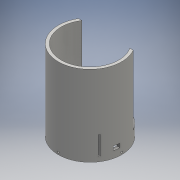
# Autodesk Inventor part: outsideCover
Saved by Autodesk Inventor 2016 (Build 200138000, 138)
## iProperties
Created: 2016-10-27
Part Number: outsideCover
Material: 一般
Document SubType Name: Modeling
Designer: Daisuke
Density: 1 g/cm^3
Appearance: 既定
Author: Daisuke
Autodesk Inventor part; units mm, degrees
ref_plane "XY Plane" through (0, 0, 0) normal (0, 0, 1) x (1, 0, 0)
sketch "スケッチ1" plane through (0, 0, 0) normal (0, 0, 1) x (1, 0, 0)
  circle A0 centre (0, 0) radius 50
  circle A1 centre (0, 0) radius 55
  line L0 (0, 0) -> (47.6314, 27.5) construction
  line L1 (0, 0) -> (55, 0) construction
  line L2 (0, 0) -> (-47.6314, 27.5) construction
  line L3 (0, 0) -> (55, 0) construction
  dimension "d0" = 100
  dimension "d1" = 110
  dimension "d2" = 30
  dimension "d3" = 150
  constraints: 8 end point, 2 centre point, 2 coincident, 2 equal length, 2 horizontal, 2 point on circle
  measures "d0" diameter of A0
  measures "d1" diameter of A1
  measures "d2" angle of L1 L0
  measures "d3" angle of L3 L2
extrude "押し出し1" add sketch "スケッチ1" along normal blind 20
sketch "スケッチ2" plane through (0, 0, 20) normal (0, 0, 1) x (1, 0, 0)
  arc A0 (-41.7582, 27.5) -> (41.7582, 27.5) centre (0, 0) ccw
  arc A1 (-47.6314, 27.5) -> (47.6314, 27.5) centre (0, 0) ccw
  line L0 (0, 0) -> (47.6314, 27.5) construction
  circle A2 centre (0, 0) radius 55 construction
  line L1 (0, 0) -> (55, 0) construction
  line L2 (0, 0) -> (-47.6314, 27.5) construction
  line L3 (0, 0) -> (55, 0) construction
  line L4 (-47.6314, 27.5) -> (-41.7582, 27.5)
  line L5 (41.7582, 27.5) -> (47.6314, 27.5)
  dimension "d6" = 30
  dimension "d7" = 150
  constraints: 12 end point, 6 point on circle, 2 centre point, 2 coincident, 2 equal length, 2 horizontal
  measures "d6" angle of L1 L0
  measures "d7" angle of L3 L2
extrude "押し出し2" add sketch "スケッチ2" along normal blind 120
ref_plane "作業平面1" through (55, 0, 0) normal (1, 0, 0) x (0, 1, 0)
ref_plane "作業平面2" through (-55, 0, 0) normal (1, 0, 0) x (0, 1, 0)
ref_plane "作業平面3" through (0, 55, 0) normal (0, 1, 0) x (-1, 0, 0)
ref_plane "作業平面4" through (0, -55, 0) normal (0, 1, 0) x (-1, 0, 0)
sketch "スケッチ3" plane through (55, 0, 0) normal (1, 0, 0) x (0, 1, 0)
  line L0 (0, 0) -> (0, 4) construction
  circle A0 centre (0, 4) radius 1.5
  dimension "d14" = 4
  dimension "d15" = 3
  constraints: 2 end point, 1 centre point, 1 coincident, 1 vertical
  measures "d14" distance of L0.start L0.end
  measures "d15" diameter of A0
extrude "押し出し3" cut sketch "スケッチ3" against normal blind 6
sketch "スケッチ4" plane through (0, 55, 0) normal (0, 1, 0) x (-1, 0, 0)
  line L0 (0, 0) -> (0, 4) construction
  circle A0 centre (0, 4) radius 1.5
  dimension "d18" = 4
  dimension "d19" = 3
  constraints: 2 end point, 1 centre point, 1 coincident, 1 vertical
  measures "d18" distance of L0.start L0.end
  measures "d19" diameter of A0
extrude "押し出し4" cut sketch "スケッチ4" against normal blind 6
sketch "スケッチ5" plane through (-55, 0, 0) normal (1, 0, 0) x (0, 1, 0)
  line L0 (0, 0) -> (0, 4) construction
  circle A0 centre (0, 4) radius 1.5
  dimension "d22" = 4
  dimension "d23" = 3
  constraints: 2 end point, 1 centre point, 1 coincident, 1 vertical
  measures "d22" distance of L0.start L0.end
  measures "d23" diameter of A0
extrude "押し出し5" cut sketch "スケッチ5" along normal blind 6
sketch "スケッチ6" plane through (0, -55, 0) normal (0, 1, 0) x (-1, 0, 0)
  line L0 (0, 0) -> (0, 4) construction
  circle A0 centre (0, 4) radius 1.5
  dimension "d26" = 4
  dimension "d27" = 3
  constraints: 2 end point, 1 centre point, 1 coincident, 1 vertical
  measures "d26" distance of L0.start L0.end
  measures "d27" diameter of A0
extrude "押し出し6" cut sketch "スケッチ6" along normal blind 6
ref_plane "作業平面5" through (55, 0, 0) normal (1, 0, 0) x (0, 1, 0)
sketch "スケッチ7" plane through (55, 0, 0) normal (1, 0, 0) x (0, 1, 0)
  line L0 (0, 0) -> (0, 12) construction
  line L1 (0, 12) -> (-3, 12) construction
  line L2 (-3, 12) -> (-13, 12)
  line L3 (-13, 12) -> (-13, 19)
  line L4 (-13, 19) -> (-3, 19)
  line L5 (-3, 19) -> (-3, 12)
  line L6 (0, 0) -> (0, 8) construction
  line L7 (0, 8) -> (-31, 8) construction
  line L8 (-31, 8) -> (-28.5, 8)
  line L9 (-28.5, 8) -> (-28.5, 41)
  line L10 (-28.5, 41) -> (-31, 41)
  line L11 (-31, 41) -> (-31, 8)
  dimension "d31" = 12
  dimension "d32" = 3
  dimension "d33" = 10
  dimension "d34" = 7
  dimension "d37" = 8
  dimension "d38" = 31
  dimension "d39" = 2.5
  dimension "d40" = 33
  constraints: 24 end point, 4 parallel, 3 horizontal, 3 perpendicular, 1 point on line, 1 vertical
  measures "d31" distance of L0.start L0.end
  measures "d32" distance of L0.end L1.end
  measures "d33" distance of L3.end L4.end
  measures "d34" distance of L4.end L1.end
  measures "d37" distance of L0.start L6.end
  measures "d38" distance of L6.end L7.end
  measures "d39" distance of L10.end L9.end
  measures "d40" distance of L9.end L8.end
extrude "押し出し8" cut sketch "スケッチ7" against normal blind 20
